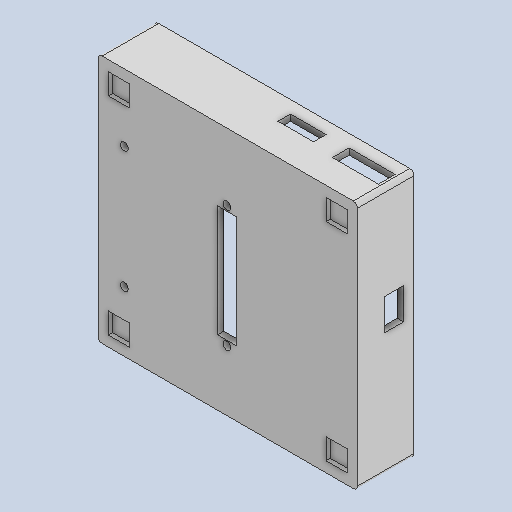
# Autodesk Inventor part: coque_RPI
Saved by Autodesk Inventor 2023 (Build 270158000, 158)
## iProperties
Created: 2023-03-27
Part Number: coque_RPI
Material: Générique
Document SubType Name: Modeling
Designer: egozi
Density: 1 g/cm^3
Appearance: Par défaut
Author: egozi
Autodesk Inventor part; units mm, degrees
ref_plane "YZ Plane" through (0, 0, 0) normal (1, 0, 0) x (0, 1, 0)
ref_plane "XZ Plane" through (0, 0, 0) normal (0, 1, 0) x (-1, 0, 0)
ref_plane "XY Plane" through (0, 0, 0) normal (0, 0, 1) x (1, 0, 0)
sketch "Esquisse1" plane through (0, 0, 0) normal (0, 0, 1) x (1, 0, 0)
  line L0 (0, -47.8) -> (0, 118.8) projected
  line L1 (-27.8, 0) -> (145.8, 0) projected
  line L2 (0, 92) -> (105, 92)
  line L3 (105, 92) -> (105, 0)
  line L4 (105, 0) -> (0, 0)
  line L5 (0, 0) -> (0, 92)
  line L6 (56.1007, 59.272) -> (61.1007, 59.272)
  line L7 (61.1007, 59.272) -> (61.1007, 8.472)
  line L8 (61.1007, 8.472) -> (56.1007, 8.472)
  line L9 (56.1007, 8.472) -> (56.1007, 59.272)
  line L10 (0, 92) -> (118, 92)
  line L11 (118, 92) -> (118, -21)
  line L12 (118, -21) -> (0, -21)
  line L13 (0, -21) -> (0, 92)
  line L14 (54.1007, 60.572) -> (63.1007, 60.572)
  line L15 (63.1007, 60.572) -> (63.1007, 7.172)
  line L16 (63.1007, 7.172) -> (54.1007, 7.172)
  line L17 (54.1007, 7.172) -> (54.1007, 60.572)
  line L18 (-3, 95) -> (121, 95)
  line L19 (121, 95) -> (121, -24)
  line L20 (121, -24) -> (-3, -24)
  line L21 (-3, -24) -> (-3, 95)
  line L22 (0, 92) -> (118, 92)
  line L23 (118, 92) -> (118, -21)
  line L24 (118, -21) -> (0, -21)
  line L25 (0, -21) -> (0, 92)
  line L26 (57.2447, 8.472) -> (59.9567, 8.472) projected
  line L27 (59.9567, 59.272) -> (57.2447, 59.272) projected
  line L28 (56.1007, 33.3434) -> (56.1007, 31.8605) projected
  line L29 (61.1007, 31.8605) -> (61.1007, 33.3434) projected
  circle A0 centre (58.6009, 4.8718) radius 1.3752 projected
  circle A1 centre (58.601, 62.8718) radius 1.3753 projected
  circle A2 centre (9.6007, 62.872) radius 1.375 projected
  circle A3 centre (9.6008, 4.8721) radius 1.3752 projected
  circle A4 centre (9.6008, 4.8721) radius 1.8752
  circle A5 centre (9.6007, 62.872) radius 1.875
  circle A6 centre (58.601, 62.8718) radius 1.8753
  circle A7 centre (58.6009, 4.8718) radius 1.8752
  point P0 (0, 0)
  point P1 (58.6007, 59.272)
  dimension "d0" = 92
  dimension "d1" = 105
  dimension "d6" = 13
  dimension "d7" = 21
  dimension "d8" = 2
  dimension "d9" = 1.3
  dimension "d11" = 1.3
  dimension "d12" = 3
  dimension "d13" = 3
  dimension "d14" = 3
  dimension "d15" = 3
  dimension "d77" = 2
  dimension "d78" = 0.5
  dimension "d79" = 0.5
  dimension "d80" = 0.5
  dimension "d81" = 0.5
  constraints: 48 end point, 12 parallel, 6 collinear, 6 horizontal, 6 perpendicular, 4 centre point, 4 coincident, 1 midpoint
  measures "d0" distance between parallel lines of L4 L2
  measures "d1" distance between parallel lines of L5 L3
  measures "d6" distance between parallel lines of L3 L11
  measures "d7" distance between parallel lines of L4 L12
  measures "d8" distance between parallel lines of L9 L17
  measures "d9" distance from line of point (58.601, 59.272) L14
  measures "d11" distance between parallel lines of L8 L16
  measures "d12" distance between parallel lines of L11 L19
  measures "d13" distance between parallel lines of L5 L21
  measures "d14" distance between parallel lines of L2 L18
  measures "d15" distance between parallel lines of L12 L20
  measures "d77" distance between parallel lines of L7 L15
  measures "d78" radial gap between concentric circles of A4 A3
  measures "d79" radial gap between concentric circles of A5 A2
  measures "d80" radial gap between concentric circles of A6 A1
  measures "d81" radial gap between concentric circles of A0 A7
extrude "Extrusion1" add sketch "Esquisse1" along normal blind 4 contours L0 L20 L21 L1 | L12 L11 L1 L19 L20 L0 | L0 L1 L11 L12 | L1 L21 L18 L0 | L0 L2 L3 L1 | L0 L18 L19 L1 L11 L10 L2 | L3 L10 L11 L1
sketch "Esquisse2" plane through (0, 0, 4) normal (0, 0, 1) x (1, 0, 0)
  line L0 (-3, -24) -> (121, -24) projected
  line L1 (-3, 95) -> (121, 95)
  line L2 (121, 95) -> (121, -24)
  line L3 (121, -24) -> (-3, -24)
  line L4 (-3, -24) -> (-3, 95)
  line L5 (0, 92) -> (118, 92)
  line L6 (118, 92) -> (118, -21)
  line L7 (118, -21) -> (0, -21)
  line L8 (0, -21) -> (0, 92)
  point P0 (0, 0)
  dimension "d18" = 3
  dimension "d19" = 3
  dimension "d20" = 3
  dimension "d21" = 3
  constraints: 16 end point, 4 parallel, 2 horizontal, 2 perpendicular
  measures "d18" distance between parallel lines of L6 L2
  measures "d19" distance between parallel lines of L4 L8
  measures "d20" distance between parallel lines of L1 L5
  measures "d21" distance between parallel lines of L0 L7
extrude "Extrusion2" add sketch "Esquisse2" against normal blind 27
sketch "Esquisse4" plane through (-3, -24, 4) normal (0, -1, 0) x (1, 0, 0)
  line L0 (27.38, -19.5) -> (27.38, -6) construction
  line L1 (27.38, -6) -> (11.5, -6) construction
  line L2 (11.5, -6) -> (11.5, -19.5) construction
  line L3 (62.1007, -19.5) -> (12.1007, -19.5) construction
  line L4 (9.1005, -19.5) -> (15.101, -19.5) construction
  line L5 (41.19, -4.01) -> (35.19, -4.01) construction
  line L6 (44.5455, -4.11) -> (31.8345, -4.11) construction
  line L7 (41.19, -2.5351) -> (41.19, -5.6849) construction
  line L8 (35.19, -5.6849) -> (35.19, -2.5351) construction
  circle A0 centre (31.94, -4.51) radius 0.4 construction
  line L9 (31.54, -4.4044) -> (31.54, -9.4204) construction
  line L10 (31.3, -5.5007) -> (31.3, -19.2199) construction
  line L11 (31.3, -5.3465) -> (31.3, -5.5636) construction
  line L12 (31.7209, -4.66) -> (31.5122, -4.66) construction
  line L13 (31.7172, -4.66) -> (31.5053, -4.66) construction
  line L14 (30.64, -9.7204) -> (30.64, -12.7204) construction
  line L15 (30.64, -12.7204) -> (31.3599, -12.7204) construction
  line L16 (31.322, -9.7204) -> (30.64, -9.7204) construction
  line L17 (44.44, -9.27) -> (44.44, -14.39) construction
  line L18 (63.74, -12.7204) -> (63.74, -9.7204) construction
  line L19 (63.08, -19.182) -> (63.08, -5.5251) construction
  line L20 (60.2447, -19.5) -> (62.9567, -19.5) construction
  line L21 (63.08, -18.9857) -> (63.08, -19.517) construction
  line L22 (59.1017, -19.5) -> (65.1003, -19.5) construction
  line L23 (63.08, -4.6635) -> (63.08, -6.647) construction
  circle A1 centre (62.4398, -4.5101) radius 0.4002 construction
  line L24 (62.84, -9.4204) -> (62.84, -4.4044) construction
  line L25 (62.8795, -4.66) -> (62.5088, -4.66) construction
  line L26 (63.08, -4.6726) -> (63.08, -4.66) construction
  line L27 (62.5455, -4.11) -> (49.8345, -4.11) construction
  circle A2 centre (49.94, -4.51) radius 0.4 construction
  line L28 (49.54, -4.4044) -> (49.54, -9.4204) construction
  line L29 (64.08, -20) -> (48.54, -20)
  line L30 (48.54, -20) -> (48.54, -3.61)
  line L31 (48.54, -3.61) -> (64.08, -3.61)
  line L32 (64.08, -3.61) -> (64.08, -20)
  line L33 (45.88, -20) -> (30.3, -20)
  line L34 (30.3, -20) -> (30.3, -3.61)
  line L35 (30.3, -3.61) -> (45.88, -3.61)
  line L36 (45.88, -3.61) -> (45.88, -20)
  line L37 (44.88, -5.5659) -> (44.88, -19.1471) projected
  line L38 (27.88, -20) -> (11, -20) construction
  line L39 (11, -20) -> (11, -5.5) construction
  line L40 (11, -5.5) -> (27.88, -5.5) construction
  line L41 (27.88, -5.5) -> (27.88, -20) construction
  line L42 (27.88, -20) -> (11, -20)
  line L43 (11, -20) -> (11, -5.5)
  line L44 (11, -5.5) -> (27.88, -5.5)
  line L45 (27.88, -5.5) -> (27.88, -20)
  point P0 (3, -4)
  dimension "d52" = 0.5
  dimension "d53" = 1
  dimension "d54" = 0.5
  dimension "d55" = 1
  dimension "d56" = 1
  dimension "d57" = 1
  dimension "d59" = 0.5
  dimension "d60" = 0.5
  dimension "d61" = 0.5
  dimension "d62" = 0.5
  dimension "d63" = 0.5
  dimension "d64" = 0.5
  constraints: 32 end point, 8 parallel, 4 horizontal, 4 perpendicular
  measures "d52" distance between parallel lines of L3 L29
  measures "d53" distance between parallel lines of L19 L32
  measures "d54" distance between parallel lines of L27 L31
  measures "d55" distance between parallel lines of L28 L30
  measures "d56" distance between parallel lines of L36 L37
  measures "d57" distance between parallel lines of L34 L10
  measures "d59" distance between parallel lines of L35 L6
  measures "d60" distance between parallel lines of L33 L3
  measures "d61" distance between parallel lines of L3 L38
  measures "d62" distance between parallel lines of L2 L39
  measures "d63" distance between parallel lines of L1 L40
  measures "d64" distance between parallel lines of L0 L41
extrude "Extrusion4" cut sketch "Esquisse4" against normal blind 27
sketch "Esquisse5" plane through (-3, -24, 4) normal (-1, 0, 0) x (0, 0, 1)
  line L0 (-13.62, 51.6049) -> (-13.62, 65.2689) projected
  line L1 (-19.17, 63.3546) -> (-19.17, 58.0099) projected
  line L2 (-19.17, 57.98) -> (-19.17, 53.5054) projected
  line L3 (-16.9746, 76.7653) -> (-16.9746, 82.8881) projected
  line L4 (-19.7386, 82.3643) -> (-19.7386, 79.9819) projected
  line L5 (-19.7386, 79.6728) -> (-19.7386, 77.3076) projected
  line L6 (-17.0251, 50.93) -> (-14.2949, 50.93) projected
  line L7 (-14.2811, 65.93) -> (-17.0251, 65.93) projected
  line L8 (-18.2776, 75.8396) -> (-17.9619, 75.8396) projected
  line L9 (-17.9553, 83.8204) -> (-18.271, 83.8204) projected
  line L10 (-22.395, 47.43) -> (-10.395, 47.43)
  line L11 (-10.395, 47.43) -> (-10.395, 69.43)
  line L12 (-10.395, 69.43) -> (-22.395, 69.43)
  line L13 (-22.395, 69.43) -> (-22.395, 47.43)
  line L14 (-22.3566, 72.8396) -> (-14.3566, 72.8396)
  line L15 (-14.3566, 72.8396) -> (-14.3566, 86.8396)
  line L16 (-14.3566, 86.8396) -> (-22.3566, 86.8396)
  line L17 (-22.3566, 86.8396) -> (-22.3566, 72.8396)
  point P0 (-4, 24)
  point P1 (-16.395, 69.43)
  point P2 (-18.1197, 75.8396)
  dimension "d67" = 22
  dimension "d68" = 12
  dimension "d69" = 3.225
  dimension "d70" = 3.5
  dimension "d71" = 14
  dimension "d72" = 8
  dimension "d73" = 2.618
  dimension "d74" = 3
  constraints: 16 end point, 4 parallel, 2 horizontal, 2 midpoint, 2 perpendicular
  measures "d67" distance of L10.end L11.end
  measures "d68" distance between parallel lines of L11 L13
  measures "d69" distance between parallel lines of L13 L1
  measures "d70" distance from line of point (-16.395, 69.43) L7
  measures "d71" distance of L16.end L14.start
  measures "d72" distance of L15.end L16.end
  measures "d73" distance between parallel lines of L15 L3
  measures "d74" distance from line of L14 point (-18.12, 75.84)
extrude "Extrusion5" cut sketch "Esquisse5" against normal blind 27
sketch "Esquisse6" plane through (-3, 95, 4) normal (0, 1, 0) x (1, 0, 0)
  line L0 (121, 4) -> (121, 27) projected
  line L1 (121, 27) -> (121, 0)
  line L2 (124, 0) -> (0, 0) projected
  line L3 (3, 4) -> (121, 4) projected
  line L4 (121, 4) -> (71, 4)
  line L5 (71, 4) -> (71, 21)
  line L6 (71, 21) -> (121, 21)
  line L7 (121, 21) -> (121, 4)
  line L8 (71, 21) -> (88, 21)
  line L9 (88, 21) -> (88, 15)
  line L10 (88, 15) -> (71, 15)
  line L11 (71, 15) -> (71, 21)
  line L12 (121, 21) -> (99, 21)
  line L13 (99, 21) -> (99, 13)
  line L14 (99, 13) -> (121, 13)
  line L15 (121, 13) -> (121, 21)
  point P0 (71, 12.5)
  point P1 (99, 21)
  point P2 (88, 21)
  dimension "d82" = 50
  dimension "d83" = 17
  dimension "d84" = 8
  dimension "d85" = 22
  dimension "d86" = 17
  dimension "d87" = 6
  constraints: 26 end point, 6 parallel, 3 horizontal, 3 perpendicular, 1 midpoint, 1 point on line, 1 vertical
  measures "d82" distance from line of point (71, 12.5) L0
  measures "d83" distance of L4.end L5.end
  measures "d84" distance of L12.end L13.end
  measures "d85" distance of L13.end L14.end
  measures "d86" distance of L9.end L10.end
  measures "d87" distance of L8.end L9.end
extrude "Extrusion6" cut sketch "Esquisse6" against normal blind 3 contours L14 L13 L6 L0 | L5 L6 L9 L10
sketch "Esquisse7" plane through (121, -24, 4) normal (1, 0, 0) x (0, 0, -1)
  line L0 (22, 74) -> (13, 74)
  line L1 (13, 59) -> (22, 59)
  line L2 (22, 59) -> (22, 74)
  line L3 (0, 119) -> (27, 119) projected
  line L4 (13, 74) -> (13, 59)
  line L5 (0, 0) -> (0, 119) projected
  point P0 (4, 24)
  point P1 (13, 66.5)
  dimension "d90" = 60
  dimension "d91" = 45
  dimension "d92" = 13
  dimension "d93" = 9
  constraints: 8 end point, 1 horizontal, 1 midpoint, 1 parallel
  measures "d90" distance between parallel lines of L1 L3
  measures "d91" distance between parallel lines of L3 L0
  measures "d92" distance from line of L5 point (13, 66.5)
  measures "d93" distance of L1.start L1.end
extrude "Extrusion7" cut sketch "Esquisse7" against normal blind 3
sketch "Esquisse8" plane through (0, 0, -23) normal (0, 0, -1) x (-1, 0, 0)
  line L0 (-1.5, 90.5) -> (1.5, 90.5)
  line L1 (1.5, 90.5) -> (1.5, 93.5)
  line L2 (1.5, 93.5) -> (-1.5, 93.5)
  line L3 (-1.5, 93.5) -> (-1.5, 90.5)
  line L4 (-118, 92) -> (0, 92) projected
  line L5 (-1.5, 90.5) -> (1.5, 93.5) construction
  line L6 (1.5, 90.5) -> (-1.5, 93.5) construction
  line L7 (-1.5, -19.5) -> (1.5, -19.5)
  line L8 (1.5, -19.5) -> (1.5, -22.5)
  line L9 (1.5, -22.5) -> (-1.5, -22.5)
  line L10 (-1.5, -22.5) -> (-1.5, -19.5)
  line L11 (-1.5, -19.5) -> (1.5, -22.5) construction
  line L12 (1.5, -19.5) -> (-1.5, -22.5) construction
  line L13 (-116.5, 93.5) -> (-119.5, 93.5)
  line L14 (-119.5, 93.5) -> (-119.5, 90.5)
  line L15 (-119.5, 90.5) -> (-116.5, 90.5)
  line L16 (-116.5, 90.5) -> (-116.5, 93.5)
  line L17 (-118, -21) -> (-118, 92) projected
  line L18 (-116.5, 93.5) -> (-119.5, 90.5) construction
  line L19 (-119.5, 93.5) -> (-116.5, 90.5) construction
  line L20 (-119.5, -19.5) -> (-116.5, -19.5)
  line L21 (-116.5, -19.5) -> (-116.5, -22.5)
  line L22 (-116.5, -22.5) -> (-119.5, -22.5)
  line L23 (-119.5, -22.5) -> (-119.5, -19.5)
  line L24 (-119.5, -19.5) -> (-116.5, -22.5) construction
  line L25 (-116.5, -19.5) -> (-119.5, -22.5) construction
  line L26 (1.5, 93.5) -> (-13.5, 93.5)
  line L27 (-13.5, 93.5) -> (-13.5, 78.5)
  line L28 (-13.5, 78.5) -> (1.5, 78.5)
  line L29 (1.5, 78.5) -> (1.5, 93.5)
  line L30 (1.5, -22.5) -> (-13.5, -22.5)
  line L31 (-13.5, -22.5) -> (-13.5, -7.5)
  line L32 (-13.5, -7.5) -> (1.5, -7.5)
  line L33 (1.5, -7.5) -> (1.5, -22.5)
  line L34 (-119.5, -22.5) -> (-104.5, -22.5)
  line L35 (-104.5, -22.5) -> (-104.5, -7.5)
  line L36 (-104.5, -7.5) -> (-119.5, -7.5)
  line L37 (-119.5, -7.5) -> (-119.5, -22.5)
  line L38 (-119.5, 93.5) -> (-104.5, 93.5)
  line L39 (-104.5, 93.5) -> (-104.5, 78.5)
  line L40 (-104.5, 78.5) -> (-119.5, 78.5)
  line L41 (-119.5, 78.5) -> (-119.5, 93.5)
  point P0 (0, 0)
  point P1 (0, -21)
  point P2 (-118, 78.5)
  point P3 (-104.5, 92)
  point P4 (-116.5, 92)
  point P5 (-118, 90.5)
  point P6 (-118, -7.5)
  point P7 (-118, -19.5)
  point P8 (1.5, 90.5)
  point P9 (-1.5, 92)
  point P10 (-13.5, 92)
  point P11 (-1.5, 93.5)
  dimension "d96" = 3
  dimension "d97" = 3
  dimension "d98" = 3
  dimension "d99" = 3
  dimension "d100" = 3
  dimension "d101" = 3
  dimension "d102" = 3
  dimension "d105" = 15
  dimension "d106" = 15
  dimension "d107" = 15
  dimension "d108" = 15
  dimension "d109" = 15
  constraints: 80 end point, 16 parallel, 8 horizontal, 8 midpoint, 8 perpendicular, 4 point on line
  measures "d96" distance of L0.end L1.end
  measures "d97" distance of L0.start L0.end
  measures "d98" distance of L7.end L8.end
  measures "d99" distance of L8.end L9.end
  measures "d100" distance of L21.end L22.end
  measures "d101" distance of L14.end L15.end
  measures "d102" distance of L13.end L14.end
  measures "d105" distance of L39.end L40.end
  measures "d106" distance of L35.end L36.end
  measures "d107" distance of L34.end L35.end
  measures "d108" distance of L30.end L31.end
  measures "d109" distance of L31.end L32.end
extrude "Extrusion8" cut sketch "Esquisse8" against normal blind 5
sketch "Esquisse10" plane through (0, 0, 0) normal (0, 0, -1) x (-1, 0, 0)
  line L0 (0, -21) -> (0, -7.5) projected
  line L1 (0, -21) -> (-4, -21)
  line L2 (-4, -21) -> (-4, -17)
  line L3 (-4, -17) -> (0, -17)
  line L4 (0, -17) -> (0, -21)
  line L5 (-118, -21) -> (-61.08, -21) projected
  line L6 (-118, -21) -> (-114, -21)
  line L7 (-114, -21) -> (-114, -17)
  line L8 (-114, -17) -> (-118, -17)
  line L9 (-118, -17) -> (-118, -21)
  line L10 (0, -21) -> (0, 92) projected
  line L11 (0, 92) -> (-4, 92)
  line L12 (-4, 92) -> (-4, 88)
  line L13 (-4, 88) -> (0, 88)
  line L14 (0, 88) -> (0, 92)
  line L15 (-118, 92) -> (-118, -21) projected
  line L16 (-118, 92) -> (-114, 92)
  line L17 (-114, 92) -> (-114, 88)
  line L18 (-114, 88) -> (-118, 88)
  line L19 (-118, 88) -> (-118, 92)
  line L20 (0, -21) -> (-118, -21)
  line L21 (-118, -21) -> (-118, 92)
  line L22 (-118, 92) -> (0, 92)
  line L23 (0, 92) -> (0, -21)
  point P0 (0, 0)
  point P1 (0, -17)
  dimension "d119" = 4
  dimension "d120" = 4
  dimension "d121" = 4
  dimension "d122" = 4
  dimension "d123" = 4
  dimension "d124" = 4
  dimension "d125" = 4
  dimension "d126" = 4
  constraints: 40 end point, 10 parallel, 5 horizontal, 5 perpendicular
  measures "d119" distance of L1.end L2.end
  measures "d120" distance of L2.end L3.end
  measures "d121" distance of L6.end L7.end
  measures "d122" distance of L7.end L8.end
  measures "d123" distance of L12.end L13.end
  measures "d124" distance of L11.end L12.end
  measures "d125" distance of L17.end L18.end
  measures "d126" distance of L16.end L17.end
extrude "Extrusion10" cut sketch "Esquisse10" against normal blind 1 contours L3 L2 L20 L5 L7 L8 L15 L18 L17 L22 L12 L13 L10 L0
fillet "Congé1" radius 2 4 edges at (-3, -24, -9.5) (121, -24, -9.5) (-3, 95, -9.5) (121, 95, -9.5)
sketch "Esquisse11" plane through (0, 0, 4) normal (0, 0, 1) x (1, 0, 0)
  line L0 (106, 80) -> (116, 80)
  line L1 (116, 80) -> (116, 90)
  line L2 (116, 90) -> (106, 90)
  line L3 (106, 90) -> (106, 80)
  line L4 (119, 95) -> (-1, 95) projected
  line L5 (121, -22) -> (121, 93) projected
  line L6 (116, -19) -> (106, -19)
  line L7 (106, -19) -> (106, -9)
  line L8 (106, -9) -> (116, -9)
  line L9 (116, -9) -> (116, -19)
  line L10 (-1, -24) -> (119, -24) projected
  line L11 (12, -9) -> (2, -9)
  line L12 (2, -9) -> (2, -19)
  line L13 (2, -19) -> (12, -19)
  line L14 (12, -19) -> (12, -9)
  line L15 (-3, 93) -> (-3, -22) projected
  line L16 (12, 90) -> (2, 90)
  line L17 (2, 90) -> (2, 80)
  line L18 (2, 80) -> (12, 80)
  line L19 (12, 80) -> (12, 90)
  point P0 (0, 0)
  point P1 (111, 90)
  point P2 (111, -19)
  dimension "d130" = 10
  dimension "d131" = 10
  dimension "d132" = 5
  dimension "d133" = 5
  dimension "d134" = 10
  dimension "d135" = 10
  dimension "d136" = 5
  dimension "d137" = 5
  dimension "d138" = 10
  dimension "d139" = 10
  dimension "d140" = 5
  dimension "d141" = 5
  dimension "d142" = 5
  dimension "d143" = 10
  dimension "d144" = 10
  dimension "d145" = 5
  constraints: 32 end point, 8 parallel, 4 horizontal, 4 perpendicular, 2 midpoint
  measures "d130" distance of L0.start L0.end
  measures "d131" distance of L2.end L0.start
  measures "d132" distance from line of L4 point (111, 90)
  measures "d133" distance between parallel lines of L5 L1
  measures "d134" distance of L7.end L8.end
  measures "d135" distance of L8.end L6.start
  measures "d136" distance from line of L10 point (111, -19)
  measures "d137" distance between parallel lines of L5 L9
  measures "d138" distance of L12.end L13.end
  measures "d139" distance of L11.end L12.end
  measures "d140" distance between parallel lines of L10 L13
  measures "d141" distance between parallel lines of L15 L12
  measures "d142" distance between parallel lines of L15 L17
  measures "d143" distance of L17.end L18.end
  measures "d144" distance of L18.end L16.start
  measures "d145" distance between parallel lines of L4 L16
extrude "Extrusion11" cut sketch "Esquisse11" against normal blind 2
